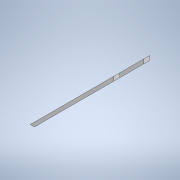
# Autodesk Inventor part: BallRamp
Saved by Autodesk Inventor 2022.2 (Build 262287000, 287)
## iProperties
Created: 2022-01-08
Part Number: BallRamp
Material: Generic
Document SubType Name: Modeling
Designer: robst
Density: 1 g/cm^3
Appearance: Default
Author: robst
Autodesk Inventor part; units mm, degrees
ref_plane "YZ Plane" through (0, 0, 0) normal (1, 0, 0) x (0, 1, 0)
ref_plane "XZ Plane" through (0, 0, 0) normal (0, 1, 0) x (-1, 0, 0)
sketch "Sketch1" plane through (0, 0, 0) normal (0, 0, 1) x (1, 0, 0)
  line L0 (0, 0) -> (711.2, 711.2)
  line L1 (0, 0) -> (1005.7887, 0) construction
  line L2 (711.2, 711.2) -> (711.2, 0) construction
  line L3 (711.2, 0) -> (0, 0) construction
  line L4 (35.921, 0) -> (711.2, 675.279)
  line L5 (0, 0) -> (35.921, 0)
  line L6 (711.2, 711.2) -> (711.2, 675.279)
  dimension "d0" = 45
  dimension "d1" = 711.2
  dimension "d2" = 25.4
  constraints: 14 end point, 3 point on line, 2 horizontal, 1 collinear, 1 equal length, 1 parallel, 1 perpendicular
  measures "d0" angle of L1 L0
  measures "d1" distance from line of L0.start L2
  measures "d2" distance between parallel lines of L4 L0
extrude "Extrusion1" add sketch "Sketch1" along normal blind 50.8
ref_plane "Work Plane1" through (0, 0, -101.6) normal (0, 0, 1) x (1, 0, 0)
mirror "Mirror1" about plane through (0, 0, -101.6) normal (0, 0, 1) of "Extrusion1"
body "Solid1"
